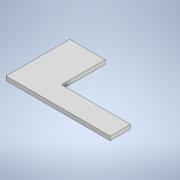
# Autodesk Inventor part: s5
Saved by Autodesk Inventor 2020 (Build 240168000, 168)
## iProperties
Created: 2019-06-28
Part Number: s5
Material: Ogólny
Document SubType Name: Modeling
Designer: atmat
Density: 1 g/cm^3
Appearance: Domyślna
Author: atmat
Autodesk Inventor part; units mm, degrees
ref_plane "YZ Plane" through (0, 0, 0) normal (1, 0, 0) x (0, 1, 0)
ref_plane "XZ Plane" through (0, 0, 0) normal (0, 1, 0) x (-1, 0, 0)
ref_plane "XY Plane" through (0, 0, 0) normal (0, 0, 1) x (1, 0, 0)
sketch "Szkic1" plane through (0, 0, 0) normal (0, 1, 0) x (-1, 0, 0)
  line L0 (10.8106, 17.9212) -> (-24.1894, 17.9212)
  line L1 (-24.1894, 17.9212) -> (-24.1894, -45.0788)
  line L2 (-24.1894, -45.0788) -> (10.8106, -45.0788)
  line L3 (10.8106, -45.0788) -> (10.8106, 17.9212)
  line L4 (10.8106, 17.9212) -> (-92.1894, 17.9212)
  line L5 (-92.1894, 17.9212) -> (-92.1894, -2.0788)
  line L6 (-92.1894, -2.0788) -> (10.8106, -2.0788)
  line L7 (10.8106, -2.0788) -> (10.8106, 17.9212)
  point P0 (0, 0)
  point P1 (-24.1894, -2.0788)
  dimension "d0" = 35
  dimension "d1" = 63
  dimension "d2" = 20
  dimension "d3" = 103
  constraints: 16 end point, 4 parallel, 2 horizontal, 2 perpendicular
  measures "d0" distance of L0.start L0.end
  measures "d1" distance of L2.end L0.start
  measures "d2" distance of L4.end L5.end
  measures "d3" distance between parallel lines of L3 L5
extrude "Wyciągnięcie proste1" add sketch "Szkic1" along normal blind 4
